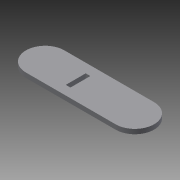
# Autodesk Inventor part: arm-servo
Saved by Autodesk Inventor 2013 (Build 170138000, 138)
## iProperties
Created: 2012-09-08
Part Number: arm-servo
Material: Generic
Document SubType Name: Modeling
Designer: frankenteddy
Density: 1 g/cm^3
Author: frankenteddy
Autodesk Inventor part; units mm, degrees
ref_plane "YZ Plane" through (0, 0, 0) normal (1, 0, 0) x (0, 1, 0)
ref_plane "XZ Plane" through (0, 0, 0) normal (0, 1, 0) x (-1, 0, 0)
ref_plane "XY Plane" through (0, 0, 0) normal (0, 0, 1) x (1, 0, 0)
sketch "Block1" plane through (0, 0, 0) normal (0, 0, 1) x (1, 0, 0)
  circle A0 centre (74.029, 24.2723) radius 1
  line L0 (49.279, 30.4723) -> (71.779, 30.4723)
  line L1 (71.779, 30.4723) -> (71.779, 18.0723)
  line L2 (71.779, 18.0723) -> (49.279, 18.0723)
  line L3 (49.279, 18.0723) -> (49.279, 30.4723)
  line L4 (49.279, 30.4723) -> (44.779, 30.4723)
  line L5 (44.779, 30.4723) -> (44.779, 18.0723)
  line L6 (44.779, 18.0723) -> (49.279, 18.0723)
  line L7 (49.279, 18.0723) -> (49.279, 30.4723)
  line L8 (71.779, 30.4723) -> (76.279, 30.4723)
  line L9 (76.279, 30.4723) -> (76.279, 18.0723)
  line L10 (76.279, 18.0723) -> (71.779, 18.0723)
  line L11 (71.779, 18.0723) -> (71.779, 30.4723)
  line L12 (44.779, 24.2723) -> (76.279, 24.2723) construction
  line L13 (47.029, 30.4723) -> (47.029, 18.0723) construction
  circle A1 centre (47.029, 24.2723) radius 1
  line L14 (74.029, 30.4723) -> (74.029, 18.0723) construction
  point P0 (60.979, 24.0984)
  dimension "d7" = 22.5
  dimension "d8" = 12.4
  dimension "d9" = 4.5
  dimension "d10" = 4.5
  dimension "d11" = 2
  dimension "d12" = 2
  measures "d7" distance of L1.end L2.end
  measures "d8" distance of L0.end L1.end
  measures "d9" distance of L6.end L5.end
  measures "d10" distance of L9.end L10.end
  measures "d11" diameter of A0
  measures "d12" diameter of A1
sketch "Sketch1" plane through (0, 0, 0) normal (0, 0, 1) x (1, 0, 0)
  line L0 (-92.7646, -8.503) -> (-89.7646, -8.503)
  line L1 (-89.7646, -8.503) -> (-89.7646, -11.753)
  line L2 (-89.7646, -11.753) -> (-92.7646, -11.753)
  line L3 (-92.7646, -11.753) -> (-92.7646, -8.503)
  line L4 (-92.7646, -21.6527) -> (-89.7646, -21.6527)
  line L5 (-89.7646, -21.6527) -> (-89.7646, -21.7527)
  line L6 (-89.7646, -21.7527) -> (-92.7646, -21.7527)
  line L7 (-92.7646, -21.7527) -> (-92.7646, -21.6527)
  line L8 (-66.3097, 47.8088) -> (23.6903, 47.8088)
  line L9 (23.6903, 47.8088) -> (23.6903, 20.8088)
  line L10 (23.6903, 20.8088) -> (-66.3097, 20.8088)
  line L11 (-66.3097, 20.8088) -> (-66.3097, 47.8088)
  line L12 (-66.3097, 34.3088) -> (23.6903, 34.3088) construction
  line L13 (-31.3097, 41.3088) -> (-28.0597, 41.3088)
  line L14 (-28.0597, 41.3088) -> (-28.0597, 27.3088)
  line L15 (-28.0597, 27.3088) -> (-31.3097, 27.3088)
  line L16 (-31.3097, 27.3088) -> (-31.3097, 41.3088)
  line L17 (-31.3097, 34.3088) -> (-28.0597, 34.3088) construction
  line L18 (-53.3097, 47.8088) -> (-53.3097, 20.8088) construction
  line L19 (-21.3097, 47.8088) -> (-21.3097, 20.8088) construction
  line L20 (10.6903, 47.8088) -> (10.6903, 20.8088) construction
  arc A0 (-53.3097, 47.8088) -> (-53.3097, 20.8088) centre (-52.8001, 34.3088) ccw
  arc A1 (10.6903, 20.8088) -> (10.6903, 47.8088) centre (10.1806, 34.3088) ccw
  point P0 (0, 0)
  dimension "d0" = 3
  dimension "mat" = 3.25
  dimension "d2" = 3
  dimension "d3" = 0.1
  dimension "d23" = 90
  dimension "d24" = 27
  dimension "d29" = 3.25
  dimension "d30" = 14
  dimension "d31" = 35
  dimension "d36" = 13
  dimension "d38" = 13
  constraints: 42 end point, 9 parallel, 6 midpoint, 6 point on circle, 5 perpendicular, 4 horizontal, 4 point on line, 2 centre point, 1 collinear
  measures "d0" distance of L1.end L3.start
  measures "mat" distance of L1.start L1.end
  measures "d2" distance of L5.end L7.start
  measures "d3" distance of L5.start L5.end
  measures "d23" distance of L9.end L10.end
  measures "d24" distance of L8.end L9.end
  measures "d29" distance of L14.end L15.end
  measures "d30" distance of L13.end L14.end
  measures "d31" distance between parallel lines of L11 L16
  measures "d36" distance between parallel lines of L11 L18
  measures "d38" distance between parallel lines of L9 L20
extrude "Extrusion5" add sketch "Sketch1" along normal blind 3.25 contours L8 A1 L10 A0
equation "\"d29\" = mat"
equation "\"d42\" = mat"
body "Solid5"
